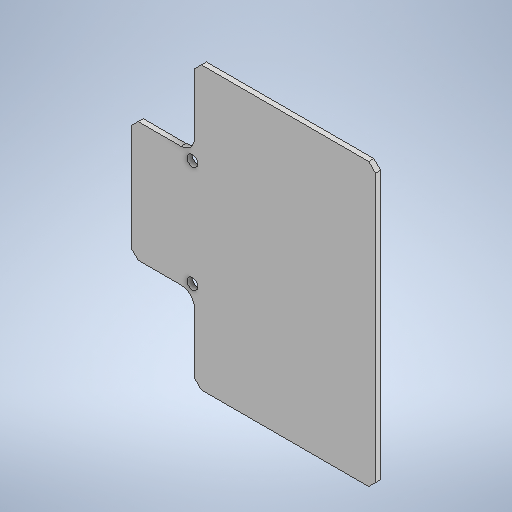
# Autodesk Inventor part: power_board
Saved by Autodesk Inventor 2025 (Build 290162000, 162)
## iProperties
Created: 2026-08-11
Part Number: power_board
Material: Типовые
Document SubType Name: Modeling
Designer: garin
Density: 1 g/cm^3
Appearance: По умолчанию
Author: garin
Autodesk Inventor part; units mm, degrees
ref_plane "YZ Plane" through (0, 0, 0) normal (1, 0, 0) x (0, 1, 0)
ref_plane "XZ Plane" through (0, 0, 0) normal (0, 1, 0) x (-1, 0, 0)
ref_plane "XY Plane" through (0, 0, 0) normal (0, 0, 1) x (1, 0, 0)
sketch "Эскиз1" plane through (0, 0, 0) normal (0, 0, 1) x (1, 0, 0)
  line L0 (-30, 41.5) -> (28, 41.5)
  line L1 (30, 39.5) -> (30, -39.5)
  line L2 (28, -41.5) -> (-30, -41.5)
  line L3 (-30, -41.5) -> (-30, 41.5)
  line L4 (-30, 41.5) -> (30, -41.5) construction
  line L5 (30, 41.5) -> (-30, -41.5) construction
  line L6 (-30, -41.5) -> (-38, -41.5)
  line L7 (-42, -37.5) -> (-42, 37.5)
  line L8 (-38, 41.5) -> (-30, 41.5)
  line L9 (-30, 41.5) -> (-30, -41.5)
  line L10 (-38, -41.5) -> (-42, -37.5)
  line L11 (-42, 37.5) -> (-38, 41.5)
  line L12 (28, 41.5) -> (30, 39.5)
  line L13 (28, -41.5) -> (30, -39.5)
  line L14 (0, 0) -> (-23.984, 0) construction
  line L15 (-23.984, 0) -> (-23.984, 15.7) construction
  line L16 (-23.984, 15.7) -> (0, 15.7) construction
  line L17 (0, 15.7) -> (0, 0) construction
  circle A0 centre (-23.984, 15.7) radius 1.6
  circle A1 centre (-23.984, -15.7) radius 1.6
  circle A2 centre (23.984, 15.7) radius 1.6
  circle A3 centre (23.984, -15.7) radius 1.6
  line L18 (-42, -41.5) -> (-23.368, -41.5)
  line L19 (-23.368, -41.5) -> (-23.368, -21.7)
  line L20 (-27.368, -17.7) -> (-42, -17.7)
  line L21 (-42, -17.7) -> (-42, -41.5)
  arc A4 (-23.368, -21.7) -> (-27.368, -17.7) centre (-27.368, -21.7) ccw
  line L22 (-23.368, 41.5) -> (-23.368, 21.7)
  line L23 (-27.368, 17.7) -> (-42, 17.7)
  arc A5 (-27.368, 17.7) -> (-23.368, 21.7) centre (-27.368, 21.7) ccw
  point P0 (-42, 41.5)
  point P1 (-23.368, -17.7)
  dimension "d0" = 60
  dimension "d1" = 83
  dimension "d2" = 12
  dimension "d3" = 83
  dimension "d6" = 4
  dimension "d7" = 4
  dimension "d8" = 4
  dimension "d9" = 4
  dimension "d10" = 2
  dimension "d11" = 2
  dimension "d12" = 2
  dimension "d13" = 2
  dimension "d14" = 23.984
  dimension "d15" = 15.7
  dimension "d16" = 3.2
  dimension "d17" = 18.632
  dimension "d18" = 23.8
  dimension "d19" = 4
  constraints: 48 end point, 10 point on line, 8 parallel, 8 symmetric about line, 6 centre point, 4 horizontal, 4 perpendicular, 4 point on circle, 2 midpoint, 2 tangent, 1 coincident, 4 other
  measures "d0" distance of L4.end L2.end
  measures "d1" distance of L5.start L4.end
  measures "d2" distance of point (-42, 41.5) L8.end
  measures "d3" distance of L18.start point (-42, 41.5)
  measures "d6" distance of L6.end L18.start
  measures "d7" distance of L7.start L18.start
  measures "d8" distance of L7.end point (-42, 41.5)
  measures "d9" distance of L8.start point (-42, 41.5)
  measures "d10" distance of L0.end L5.start
  measures "d11" distance of L1.start L5.start
  measures "d12" distance of L2.start L4.end
  measures "d13" distance of L1.end L4.end
  measures "d14" distance of L15.end L16.end
  measures "d15" distance of L14.end L15.end
  measures "d16" diameter of A0
  measures "d17" distance of L20.end point (-23.368, -17.7)
  measures "d18" distance of point (-23.368, -17.7) L18.end
  measures "d19" radius of A4
extrude "Выдавливание1" add sketch "Эскиз1" along normal blind 1.5 contours L0 L12 L1 L13 L2 L19 A4 L20 L3 L23 A5 L22 | L3 L20 L7 L23 | A2 | A3
chamfer "Фаска1" distance 2 angle 45 4 edges at (-42, -17.7, 0.75) (-42, 17.7, 0.75) (-23.368, -41.5, 0.75) (-23.368, 41.5, 0.75)
equation "\"d7\" = d6"
equation "\"d9\" = d8"
equation "\"d11\" = d10"
